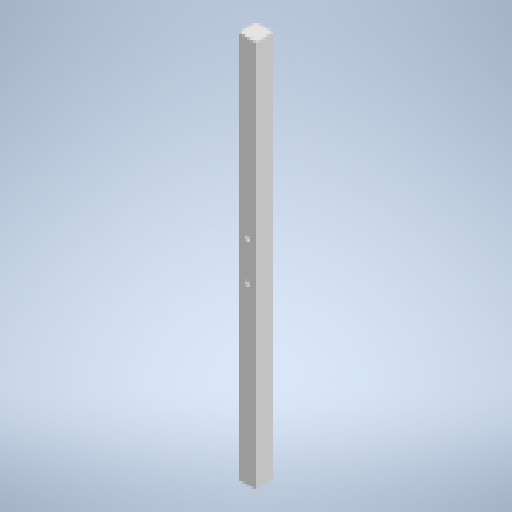
# Autodesk Inventor part: DOF3
Saved by Autodesk Inventor 2024 (Build 280153000, 153)
## iProperties
Created: 2024-10-15
Part Number: DOF3
Material: 一般
Document SubType Name: Modeling
Designer: jerry
Density: 1 g/cm^3
Appearance: 預設
Author: jerry
Autodesk Inventor part; units mm, degrees
ref_plane "YZ Plane" through (0, 0, 0) normal (1, 0, 0) x (0, 1, 0)
ref_plane "XZ Plane" through (0, 0, 0) normal (0, 1, 0) x (-1, 0, 0)
ref_plane "XY Plane" through (0, 0, 0) normal (0, 0, 1) x (1, 0, 0)
sketch "草圖1" plane through (0, 0, 0) normal (0, 0, 1) x (1, 0, 0)
  line L0 (-5, 215) -> (-25, 215)
  line L1 (-25, 215) -> (-25, -235)
  line L2 (-25, -235) -> (-5, -235)
  line L3 (-5, -235) -> (-5, 215)
  line L4 (-5, 215) -> (-25, -235) construction
  line L5 (-25, 215) -> (-5, -235) construction
  circle A0 centre (-15, 12.5) radius 3
  circle A1 centre (-15, -32.5) radius 3
  point P0 (0, 0)
  point P1 (-15, -10)
  dimension "d2" = 20
  dimension "d3" = 450
  dimension "d5" = 6
  dimension "d6" = 6
  constraints: 12 end point, 2 centre point, 2 midpoint, 2 parallel, 1 horizontal, 1 perpendicular
  measures "d2" distance of L2.end L1.end
  measures "d3" distance of L1.end L0.end
  measures "d5" diameter of A0
  measures "d6" diameter of A1
extrude "擠出1" add sketch "草圖1" along normal blind 20
